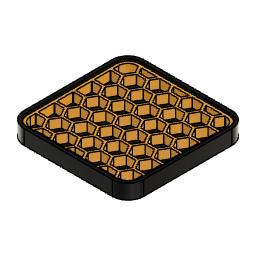
Half-Gallon Mason Jar Coaster (Autodesk Fusion 360 design; units mm, degrees)
Autodesk Fusion 360 part; units mm, degrees
note: some values were not read from the file. Chosen so that the rebuilt part matches the saved one: which bodies a step acts on.
sketch "Base" plane through (0, 0, 0) normal (0, 0, 1) x (1, 0, 0)
  line L0 (57.5, -57.5) -> (-57.5, -57.5)
  line L1 (-57.5, -57.5) -> (-57.5, 57.5)
  line L2 (-57.5, 57.5) -> (57.5, 57.5)
  line L3 (57.5, 57.5) -> (57.5, -57.5)
  line L4 (57.5, -57.5) -> (-57.5, 57.5) construction
  line L5 (-57.5, -57.5) -> (57.5, 57.5) construction
  dimension "d1" = 115
  constraint horizontal L0
  constraint perpendicular L0 L1
  constraint parallel L0 L2
  constraint parallel L1 L3
  constraint coincident L4 origin
  constraint coincident L5 origin
  constraint equal L0 L3
  measures "d1" distance of L0.start L2.end
extrude "Extrude1" add sketch "Base" along normal blind 14 makes body 1
fillet "Fillet1" radius 15 4 edges at (-57.5, -57.5, 7) (-57.5, 57.5, 7) (57.5, -57.5, 7) (57.5, 57.5, 7) on bodies 1
shell "Shell1" thickness 3 removed faces 1 at (-24.1667, -19.1667, 14) on bodies 1
sketch "Insert" plane through (0, 0, 3) normal (0, 0, 1) x (-1, 0, 0)
  arc A0 (-54.5, -42.5) -> (-42.5, -54.5) centre (-42.5, -42.5) ccw
  line L0 (-42.5, -54.5) -> (42.5, -54.5)
  arc A1 (42.5, -54.5) -> (54.5, -42.5) centre (42.5, -42.5) ccw
  line L1 (54.5, -42.5) -> (54.5, 42.5)
  arc A2 (54.5, 42.5) -> (42.5, 54.5) centre (42.5, 42.5) ccw
  line L2 (42.5, 54.5) -> (-42.5, 54.5)
  arc A3 (-42.5, 54.5) -> (-54.5, 42.5) centre (-42.5, 42.5) ccw
  line L3 (-54.5, 42.5) -> (-54.5, -42.5)
  line L4 (9, 0) -> (4.5, 7.7942)
  line L5 (4.5, 7.7942) -> (-4.5, 7.7942)
  line L6 (-4.5, 7.7942) -> (-9, 0)
  line L7 (-9, 0) -> (-4.5, -7.7942)
  line L8 (-4.5, -7.7942) -> (4.5, -7.7942)
  line L9 (4.5, -7.7942) -> (9, 0)
  line L10 (0, 0) -> (0, -34.1969)
  line L11 (0, 0) -> (-30.4783, -17.5966)
  line L12 (-51.5, 42.5) -> (-51.5, -42.5)
  arc A4 (-51.5, -42.5) -> (-42.5, -51.5) centre (-42.5, -42.5) ccw
  line L13 (-42.5, -51.5) -> (42.5, -51.5)
  arc A5 (42.5, -51.5) -> (51.5, -42.5) centre (42.5, -42.5) ccw
  line L14 (51.5, -42.5) -> (51.5, 42.5)
  arc A6 (51.5, 42.5) -> (42.5, 51.5) centre (42.5, 42.5) ccw
  line L15 (42.5, 51.5) -> (-42.5, 51.5)
  arc A7 (-42.5, 51.5) -> (-51.5, 42.5) centre (-42.5, 42.5) ccw
  line L16 (0, 0) -> (37.8096, 0)
  dimension "d10" = 9
  dimension "d17" = -3
  constraint coincident L10.start L11.start
  constraint horizontal L8
  constraint vertical L10
  constraint perpendicular L7 L11
  constraint horizontal L16
  measures "d10" distance of L4.start L8.end
extrude "Extrude2" add sketch "Insert" along normal blind 9 separate body contours A0 L0 A1 L1 A2 L2 A3 L3 | L4 L5 L6 L7 L11 L16 | L8 L9 L10 L16 | L7 L8 L10 L11 | L12 A4 L13 A5 L14 A6 L15 A7 makes body 2
move_face "OffsetFaces1" offset -0.25 8 faces at (54.5, -14.1667, 6) (51.9326, 49.9179, 9) (14.1667, 54.5, 6) (-53.166, 47.9987, 9) (-54.5, 14.1667, 6) (-47.9987, -53.166, 9) (-14.1667, -54.5, 6) (53.166, -47.9987, 9) on bodies 2
split "Split1" by curves path "Insert" along L13 A5 L14 A6 L15 A7 L12 A4 bodies 2 makes body 3 at (-14.1667, -52.4167, 3)
extrude "Extrude3" cut sketch "Insert" along normal blind 11 contours L4 L5 L6 L7 L11 L16 | L8 L9 L10 L16 | L7 L8 L10 L11 bodies 2
pattern_linear "R-Pattern1" count 7 spacing 18 along (0.866025, 0.5, 0) both ways count 9 spacing 18 along (0, 1, 0) both ways of "Extrude3"
combine "Combine1" operation add target body 3 tool bodies 2
named bodies: "Coaster Shell", "Inner-Inside", "Coaster Insert"
